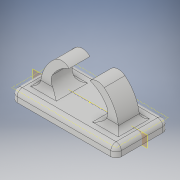
# Autodesk Inventor part: cable_holder
Saved by Autodesk Inventor 2019 (Build 230136000, 136)
## iProperties
Created: 2019-05-23
Part Number: cable_holder
Material: Generic
Document SubType Name: Modeling
Designer: assman
Density: 1 g/cm^3
Appearance: Default
Author: assman
## iProperties of the stored document cable_holder_3DPrint.ipt
Created: 2019-05-23
Part Number: cable_holder_3DPrint
Material: Generic
Document SubType Name: Modeling
Designer: assman
Density: 1 g/cm^3
Appearance: Default
Author: assman
Autodesk Inventor part; units mm, degrees
ref_plane "YZ Plane" through (0, 0, 0) normal (1, 0, 0) x (0, 1, 0)
ref_plane "XZ Plane" through (0, 0, 0) normal (0, 1, 0) x (-1, 0, 0)
ref_plane "XY Plane" through (0, 0, 0) normal (0, 0, 1) x (1, 0, 0)
sketch "Sketch1" plane through (0, 0, 0) normal (0, 1, 0) x (-1, 0, 0)
  line L0 (10, 5) -> (-10, 5)
  line L1 (-10, 5) -> (-10, -5)
  line L2 (-10, -5) -> (10, -5)
  line L3 (10, -5) -> (10, 5)
  line L4 (10, 5) -> (-10, -5) construction
  line L5 (-10, 5) -> (10, -5) construction
  point P0 (0, 0)
  dimension "d0" = 20
  dimension "d1" = 10
  constraints: 12 end point, 2 midpoint, 2 parallel, 1 horizontal, 1 perpendicular
  measures "d0" distance of L2.end L1.end
  measures "d1" distance of L1.end L0.end
extrude "Extrusion1" add sketch "Sketch1" along normal blind 2
sketch "Sketch2" plane through (0, 2, 0) normal (0, 1, 0) x (1, 0, 0)
  line L0 (-10, -5) -> (10, -5) construction
  line L1 (10, -5) -> (10, 5) construction
  line L2 (10, 5) -> (-10, 5) construction
  line L3 (-10, 5) -> (-10, -5) construction
  line L4 (-10, 5) -> (-10, -5) construction
  line L5 (-10, 0) -> (10, 0) construction
  point P0 (0, 0)
  constraints: 2 end point, 2 midpoint
ref_plane "Work Plane1" through (-10, 2, 0) normal (0, 0, 1) x (1, 0, 0)
sketch "Sketch3" plane through (-10, 2, 0) normal (0, 0, 1) x (1, 0, 0)
  line L0 (0, 0) -> (20, 0) construction
  line L1 (2.5, 0) -> (4, 0)
  line L2 (0, 0) -> (20, 0) projected
  line L3 (16, 0) -> (17.5, 0)
  arc A0 (16, 0) -> (12.0028, 5.6558) centre (10, 0) ccw
  arc A1 (7.9972, 5.6558) -> (4, 0) centre (10, 0) ccw
  arc A2 (17.5, 0) -> (12.5036, 7.0698) centre (10, 0) ccw
  arc A3 (7.4964, 7.0698) -> (2.5, 0) centre (10, 0) ccw
  line L4 (10, 0) -> (10, 7.5) construction
  line L5 (10, 0) -> (12.5036, 7.0698)
  line L6 (10, 0) -> (10, 7.5) construction
  line L7 (10, 0) -> (10, 7.5) construction
  line L8 (10, 0) -> (7.4964, 7.0698)
  line L9 (10, 0) -> (10, 7.5) construction
  point P0 (10, -2)
  point P1 (7.1395, 6.9331)
  point P2 (12.8605, 6.9331)
  point P3 (7.7742, 5.5719)
  point P4 (12.2258, 5.5719)
  point P5 (6.1541, 6.4389)
  point P6 (13.8459, 6.4389)
  dimension "d14" = 19.5
  dimension "d16" = 19.5
  constraints: 16 end point, 8 point on circle, 6 point on line, 4 centre point, 3 coincident, 2 collinear, 1 midpoint, 1 vertical
  measures "d14" angle of L5 L6
  measures "d16" angle of L9 L8
extrude "Extrusion2" add sketch "Sketch3" along normal blind 2 and the other way blind 2 contours A3 L8 A1 L1 | A0 L5 A2 L2
fillet "Fillet1" radius 2 2 edges at (-2.5036, 9.0698, 0) (2.5036, 9.0698, 0)
fillet "Fillet2" radius 1 8 edges at (0, 2, 5) (10, 2, 0) (0, 2, -5) (-10, 2, 0) (10, 1, -5) (-10, 1, -5) (-10, 1, 5) (10, 1, 5)
fillet "Fillet4" radius 2 2 edges at (-6, 2, 0) (6, 2, 0)
fillet "Fillet4" radius 1 6 edges at (6.75, 2, 2) (7.5, 2, 0) (6.75, 2, -2) (-6.75, 2, 2) (-7.5, 2, 0) (-6.75, 2, -2)
body "Solid1"
